Autodesk Fusion 360 part; units mm, degrees
(part 2 of 2)
sketch "PCB Export" plane through (0, -1.1938, 0) normal (0, -1, 0) x (1, 0, 0)
  circle A0 centre (-17.78, -45.085) radius 1.2645
  circle A1 centre (-17.78, -45.085) radius 3.175
  line L0 (-56.896, -83.8166) -> (-56.896, -47.9586)
  line L1 (-56.896, -47.9586) -> (-41.656, -47.9586)
  line L2 (-41.656, -47.9586) -> (-41.656, -83.8166)
  line L3 (-41.656, -83.8166) -> (-56.896, -83.8166)
  circle A2 centre (-17.78, -45.085) radius 3.175
  circle A3 centre (-17.78, -95.885) radius 3.175
  line L4 (-112.649, -21.6281) -> (-84.201, -21.6281)
  line L5 (-84.201, -21.6281) -> (-84.201, -110.1471)
  line L6 (-84.201, -110.1471) -> (-112.649, -110.1471)
  line L7 (-112.649, -110.1471) -> (-112.649, -21.6281)
  circle A4 centre (-49.276, -91.2876) radius 1.9685
  line L8 (-20.828, 5.2324) -> (-147.32, 5.2324)
  line L9 (-147.32, 5.2324) -> (-147.32, -137.0076)
  line L10 (-147.32, -137.0076) -> (-5.08, -137.0076)
  line L11 (-5.08, -137.0076) -> (-5.08, -3.9624)
  line L12 (-5.08, -3.9624) -> (-10.668, -3.9624)
  line L13 (-10.668, -3.9624) -> (-10.668, -2.6924)
  line L14 (-10.668, -2.6924) -> (-20.828, -2.6924)
  line L15 (-20.828, -2.6924) -> (-20.828, 5.2324)
  circle A5 centre (-98.425, -13.3731) radius 3.175
  circle A6 centre (-98.425, -118.4021) radius 3.175
  line L16 (-55.626, -49.2286) -> (-42.926, -49.2286)
  line L17 (-42.926, -49.2286) -> (-42.926, -63.9826)
  line L18 (-42.926, -63.9826) -> (-55.626, -63.9826)
  line L19 (-55.626, -63.9826) -> (-55.626, -49.2286)
  line L20 (-55.626, -82.5466) -> (-55.626, -67.7926)
  line L21 (-55.626, -67.7926) -> (-42.926, -67.7926)
  line L22 (-42.926, -67.7926) -> (-42.926, -82.5466)
  line L23 (-42.926, -82.5466) -> (-55.626, -82.5466)
  line L24 (-56.896, -83.8166) -> (-41.656, -83.8166)
  line L25 (-41.656, -83.8166) -> (-41.656, -47.9586)
  line L26 (-41.656, -47.9586) -> (-56.896, -47.9586)
  line L27 (-56.896, -47.9586) -> (-56.896, -83.8166)
  line L28 (0, -3.9624) -> (0, -137.0076)
  circle A7 centre (-49.276, -31.6281) radius 8.5
  circle A8 centre (-57.276, -39.6281) radius 0.8
  circle A9 centre (-41.276, -39.6281) radius 0.8
  circle A10 centre (-57.276, -23.6281) radius 0.8
  circle A11 centre (-41.276, -23.6281) radius 0.8
  line L29 (-39.276, -41.6281) -> (-39.276, -21.6281)
  line L30 (-39.276, -21.6281) -> (-59.276, -21.6281)
  line L31 (-59.276, -21.6281) -> (-59.276, -41.6281)
  line L32 (-59.276, -41.6281) -> (-39.276, -41.6281)
equation "d1 = 0.2 \""
equation "d4 = 0.25 \""
equation "d5 = 0.1 \""
equation "d6 = 0.05 \""
equation "d7 = 0.05 \""
equation "d9 = 0.25 \""
equation "d11 = 0.15 \""
equation "d12 = 0.15 \""
equation "d14 = 0.05 \""
equation "d15 = 0.05 \""
equation "d16 = 0.05 \""
equation "d17 = -0.10 \""
equation "d19 = 0.01 \""
equation "d20 = 0.15 \""
equation "d22 = 0.006 \""
equation "d23 = 0.27 \""
equation "d25 = 0.01 \""
equation "d26 = d25"
equation "d27 = d23"
equation "d28 = d22"
equation "d29 = d28"
equation "d31 = 6\""
equation "d32 = 0.1 \""
equation "d33 = 1\""
equation "d34 = 0.25 \""
equation "d36 = -0.26 \""
equation "d38 = 0.05 \""
equation "d39 = 0.15 \""
equation "d41 = 0.2 \""
equation "d42 = d41"
equation "d43 = d47"
equation "d45 = d41"
equation "d46 = d47"
equation "d47 = d41 / 2"
equation "d48 = d47"
equation "d49 = -0.1 \""
equation "d53 = -0.25 \""
equation "d55 = 0.1 \""
equation "d59 = d27"
equation "d60 = 0.40 \""
equation "d61 = 3.485 \""
equation "d62 = 1.12 \""
equation "d64 = 0.75 \""
equation "d65 = 1.5 \""
equation "d67 = 1\""
equation "d102 = -0.10 \""
equation "d104 = -0.05 \""
equation "d106 = 0.155 \""
equation "d107 = 0.25 \""
equation "d111 = 50 °"
equation "d112 = d111"
equation "d113 = d111"
equation "d114 = d111"
equation "d115 = 0.025 \""
equation "d116 = 0.08 \""
equation "d117 = 0.05 \""
equation "d118 = 0.25 \""
equation "d119 = 0.05 \""
equation "d120 = 135.00 °"
equation "d121 = d111"
equation "d122 = d111"
equation "d123 = 0.15 \""
equation "d124 = d111"
equation "d125 = d111"
equation "d126 = -0.05 \""
equation "d128 = 0.22 \""
equation "d129 = 0.05 \""
equation "d130 = 0.15 \""
equation "d132 = 2\""
equation "d133 = 0.5 \""
equation "d134 = 0.207 \""
equation "d136 = 0.15 \""
equation "d138 = 0.05 \""
equation "d139 = d138"
equation "d140 = d138"
equation "d141 = d138"
equation "d142 = 0.05 \""
equation "d143 = d142"
equation "d145 = 0.1 \""
equation "d147 = -0.15 \""
equation "d148 = -0.15 \""
equation "d149 = 0.07 \""
equation "d151 = 0.08 \""
equation "d157 = 0.005 \""
equation "d158 = 0.15 \""
equation "d160 = 0.09 \""
equation "d164 = ( 0.4 mm * 2 )"
equation "d165 = 0.44 mm * 4"
equation "d166 = d165"
equation "d167 = d164"
equation "d168 = d165"
equation "d169 = d167"
equation "d171 = d168"
equation "d172 = d169"
equation "d173 = d171"
equation "d174 = d164"
equation "d175 = 0.087767 \""
equation "d176 = d172"
equation "d177 = d173"
equation "d178 = d176"
equation "d179 = d177"
equation "d180 = d178"
equation "d181 = d179"
equation "d182 = d180"
equation "d183 = d181"
equation "d184 = d182"
equation "d186 = -0.05 \""
equation "d191 = 0.2 \""
equation "d192 = 0.07 \""
named bodies: "Pawl", "Top Case", "Spring Cover", "LED Defuser"
